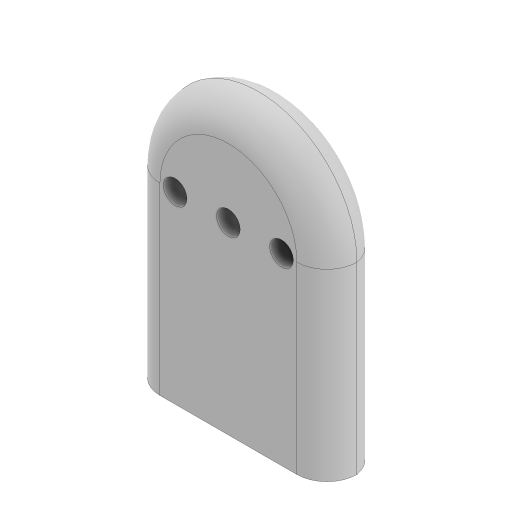
# Autodesk Inventor part: servo horn holder smoltronv2
Saved by Autodesk Inventor 2024 (Build 280153000, 153)
## iProperties
Created: 2023-09-13
Part Number: servo horn holder smoltronv2
Material: Generic
Document SubType Name: Modeling
Designer: chris
Density: 1 g/cm^3
Appearance: Default
Author: chris
Autodesk Inventor part; units mm, degrees
ref_plane "YZ Plane" through (0, 0, 0) normal (1, 0, 0) x (0, 1, 0)
ref_plane "XZ Plane" through (0, 0, 0) normal (0, 1, 0) x (-1, 0, 0)
ref_plane "XY Plane" through (0, 0, 0) normal (0, 0, 1) x (1, 0, 0)
sketch "Sketch1" plane through (0, 0, 0) normal (0, 0, 1) x (1, 0, 0)
  circle A0 centre (0, 0) radius 11
  circle A1 centre (0, 0) radius 15.875
  line L0 (-15.875, 0) -> (-15.875, -28.575)
  line L1 (-15.875, -28.575) -> (15.875, -28.575)
  line L2 (15.875, -28.575) -> (15.875, 0)
  dimension "d0" = 22
  dimension "d1" = 31.75
  dimension "d2" = 28.575
  constraints: 6 end point, 2 centre point, 2 coincident, 2 point on circle, 2 tangent, 1 perpendicular, 1 vertical
  measures "d0" diameter of A0
  measures "d1" diameter of A1
  measures "d2" distance of L0.start L0.end
extrude "Extrusion1" add sketch "Sketch1" along normal blind 7
sketch "Sketch3" plane through (-15.875, -28.575, 0) normal (0, -1, 0) x (1, 0, 0)
  line L0 (0, 7) -> (31.75, 7) projected
  line L1 (15.875, 7) -> (28.375, 7)
  line L2 (15.875, 7) -> (3.375, 7)
  line L3 (3.375, 7) -> (3.375, 55)
  line L4 (28.375, 7) -> (28.375, 55)
  line L5 (28.375, 55) -> (3.375, 55)
  point P0 (15.875, 0)
  dimension "d5" = 12.5
  dimension "d6" = 12.5
  dimension "d7" = 48
  constraints: 10 end point, 2 perpendicular, 1 collinear, 1 midpoint, 1 point on line, 1 vertical
  measures "d5" distance of L1.start L1.end
  measures "d6" distance of L1.start L2.end
  measures "d7" distance of L2.end L3.end
extrude "Extrusion2" add sketch "Sketch3" against normal blind 2.75
sketch "Sketch4" plane through (-12.5, -28.575, 55) normal (0, 0, 1) x (1, 0, 0)
  line L0 (25, 0) -> (0, 0) projected
  line L1 (25, 0) -> (25, 2.75) projected
  line L2 (0, 2.75) -> (25, 2.75) projected
  line L3 (0, 0) -> (0, 2.75) projected
  circle A0 centre (12.5, 28.575) radius 12.5
  line L4 (0, 28.575) -> (0, 0)
  line L5 (-3.375, 28.575) -> (-3.375, 0) projected
  line L6 (25, 28.575) -> (25, 0)
  line L7 (28.375, 0) -> (28.375, 28.575) projected
  point P0 (0, 2.75)
  dimension "d10" = 25
  constraints: 4 end point, 2 parallel, 2 point on circle, 1 centre point, 1 coincident
  measures "d10" diameter of A0
extrude "Extrusion3" add sketch "Sketch4" along normal blind 7
ref_plane "Work Plane1" through (-12.7, -28.575, 2.2225) normal (0, -1, 0) x (1, 0, 0)
sketch "Sketch7" plane through (0, 0, 7) normal (0, 0, 1) x (1, 0, 0)
  line L0 (-12.5, -25.825) -> (12.5, -25.825) projected
  line L1 (-12.5, -28.575) -> (-12.5, -25.825) projected
  line L2 (12.5, -25.825) -> (12.5, -28.575) projected
  line L3 (12.5, -28.575) -> (15.875, -28.575) projected
  line L4 (15.875, -28.575) -> (15.875, 0) projected
  line L5 (15.875, -25.825) -> (-19.4013, -25.825)
  circle A0 centre (0, 0) radius 11 projected
  line L6 (-12.5, -28.575) -> (-12.5, -25.825) projected
  line L7 (-12.5, -25.825) -> (12.5, -25.825) projected
  line L8 (12.5, -25.825) -> (12.5, -28.575) projected
  line L9 (12.5, -28.575) -> (15.875, -28.575) projected
  line L10 (15.875, -28.575) -> (15.875, 0) projected
  arc A1 (15.875, 0) -> (-15.875, 0) centre (0, 0) ccw projected
  line L11 (-15.875, 0) -> (-15.875, -28.575) projected
  line L12 (-15.875, -28.575) -> (-12.5, -28.575) projected
  line L13 (-15.875, -28.575) -> (-12.5, -28.575) projected
  constraints: 2 end point, 1 horizontal, 1 point on line
extrude "Extrusion7" cut sketch "Sketch7" against normal blind 25.4 fills toward (-1.7631, -25.875) open curves L5
sketch "Sketch16" plane through (-12.5, -28.575, 62) normal (0, -1, 0) x (1, 0, 0)
  line L0 (28.375, -62) -> (-3.375, -62) projected
  line L1 (28.375, -55) -> (28.375, -62) projected
  line L2 (25, -55) -> (28.375, -55) projected
  line L3 (0, -55) -> (25, -55) projected
  line L4 (-3.375, -55) -> (0, -55) projected
  line L5 (-3.375, -62) -> (-3.375, -55) projected
  line L6 (0, -55) -> (25, -55) projected
  line L7 (25, -55) -> (25, 0) projected
  line L8 (0, 0) -> (25, 0) projected
  line L9 (0, 0) -> (0, -55) projected
  point P0 (12.5, -62)
sketch "Sketch11" plane through (0, 0, 7) normal (0, 0, -1) x (-1, 0, 0)
  line L0 (-12.5, -25.825) -> (-12.5, -28.575) projected
  line L1 (12.5, -28.575) -> (-12.5, -28.575) projected
  line L2 (12.5, -28.575) -> (12.5, -25.825) projected
  line L3 (12.5, -25.825) -> (-12.5, -25.825) projected
  point P0 (0, 0)
extrude "Extrusion11" cut sketch "Sketch11" against normal through all
sketch "Sketch12" plane through (-12.5, -25.825, 55) normal (0, -1, 0) x (1, 0, 0)
  line L0 (0, 0) -> (25, 0) projected
  line L1 (25, 7) -> (25, 0) projected
  line L2 (0, 7) -> (25, 7) projected
  line L3 (0, 0) -> (0, 7) projected
  point P0 (12.5, -55)
extrude "Extrusion12" cut sketch "Sketch12" against normal blind 2.5
sketch "Sketch13" plane through (0, 0, 7) normal (0, 0, 1) x (1, 0, 0)
  line L0 (-15.875, -25.825) -> (15.875, -25.825) projected
  line L1 (15.875, -25.825) -> (15.875, 0) projected
  arc A0 (15.875, 0) -> (-15.875, 0) centre (0, 0) ccw projected
  line L2 (-15.875, 0) -> (-15.875, -25.825) projected
  circle A1 centre (0, 0) radius 11 projected
extrude "Extrusion13" cut sketch "Sketch13" against normal through all
sketch "Sketch14" plane through (-12.5, -28.575, 62) normal (0, 0, 1) x (1, 0, 0)
  circle A0 centre (12.5, 28.575) radius 1.5
  circle A1 centre (5.75, 28.575) radius 1.5
  circle A2 centre (19.25, 28.575) radius 1.5
  point P0 (12.5, 28.575)
  dimension "d54" = 3
  dimension "d55" = 3
  dimension "d56" = 3
  constraints: 3 centre point
  measures "d54" diameter of A0
  measures "d55" diameter of A1
  measures "d56" diameter of A2
extrude "Extrusion14" cut sketch "Sketch14" against normal blind 25.4
sketch "Sketch15" plane through (-12.5, -23.325, 55) normal (0, -1, 0) x (1, 0, 0)
  line L0 (140.6073, 103.7493) -> (140.6073, 110.7493)
  line L1 (124.7323, 110.7493) -> (156.4823, 110.7493)
  line L2 (140.6073, 107.2493) -> (147.5923, 107.2493)
  line L3 (140.6073, 107.2493) -> (133.6223, 107.2493)
  circle A0 centre (147.5923, 107.2493) radius 1.5
  circle A1 centre (133.6223, 107.2493) radius 1.5
  line L4 (25, 0) -> (0, 0) projected
  line L5 (12.5, 0) -> (12.5, 7)
  line L6 (25, 7) -> (0, 7) projected
  line L7 (12.5, 3.5) -> (13.5654, 3.5)
  line L8 (12.5, 0) -> (12.5, 7)
  line L9 (-3.375, 7) -> (28.375, 7)
  line L10 (12.5, 3.5) -> (19.485, 3.5)
  line L11 (12.5, 3.5) -> (5.515, 3.5)
  circle A2 centre (19.485, 3.5) radius 1.5
  circle A3 centre (5.515, 3.5) radius 1.5
  point P0 (12.5, -55)
  dimension "d59" = 6.985
  dimension "d60" = 6.985
  dimension "d61" = 3
  dimension "d62" = 3
  dimension "d63" = 6.985
  dimension "d64" = 6.985
  dimension "d65" = 3
  dimension "d66" = 3
  constraints: 20 end point, 7 midpoint, 5 horizontal, 4 centre point, 4 coincident
  measures "d59" distance of L2.start L2.end
  measures "d60" distance of L2.start L3.end
  measures "d61" diameter of A0
  measures "d62" diameter of A1
  measures "d63" distance of L10.start L10.end
  measures "d64" distance of L10.start L11.end
  measures "d65" diameter of A2
  measures "d66" diameter of A3
extrude "Extrusion15" cut sketch "Sketch15" against normal blind 15.875 contours A2 | A3
fillet "Fillet7" radius 3.81 6 edges at (-12.5, -11.6625, 62) (12.5, -11.6625, 62) (0, 12.5, 62) (-12.5, -11.6625, 55) (12.5, -11.6625, 55) (0, 12.5, 55)
body "Solid1"
